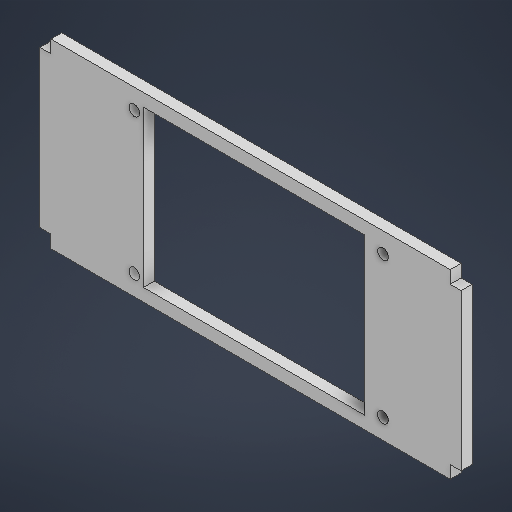
# Autodesk Inventor part: pantallaSoport
Saved by Autodesk Inventor 2026 (Build 300175000, 175)
## iProperties
Created: 2026-04-21
Part Number: pantallaSoport
Material: Generic
Document SubType Name: Modeling
Designer: juana
Density: 1 g/cm^3
Appearance: Default
Author: juana
Autodesk Inventor part; units mm, degrees
ref_plane "YZ Plane" through (0, 0, 0) normal (1, 0, 0) x (0, 1, 0)
ref_plane "XZ Plane" through (0, 0, 0) normal (0, 1, 0) x (-1, 0, 0)
ref_plane "XY Plane" through (0, 0, 0) normal (0, 0, 1) x (1, 0, 0)
sketch "Sketch1" plane through (0, 0, 0) normal (0, 0, 1) x (1, 0, 0)
  line L0 (0, 0) -> (116, 0)
  line L1 (116, 0) -> (116, 50)
  line L2 (116, 50) -> (0, 50)
  line L3 (0, 50) -> (0, 0)
  line L4 (0, 50) -> (3, 50)
  line L5 (3, 50) -> (3, 46.5)
  line L6 (3, 46.5) -> (0, 46.5)
  line L7 (0, 46.5) -> (0, 50)
  line L8 (0, 0) -> (3, 0)
  line L9 (3, 0) -> (3, 3.5)
  line L10 (3, 3.5) -> (0, 3.5)
  line L11 (0, 3.5) -> (0, 0)
  line L12 (58, 0) -> (58, 50) construction
  line L13 (113, 50) -> (113, 46.5)
  line L14 (113, 46.5) -> (116, 46.5)
  line L15 (113, 0) -> (113, 3.5)
  line L16 (113, 3.5) -> (116, 3.5)
  line L17 (19.5, 46.5) -> (96.5, 46.5) construction
  line L18 (96.5, 46.5) -> (96.5, 3.5) construction
  line L19 (96.5, 3.5) -> (19.5, 3.5) construction
  line L20 (19.5, 3.5) -> (19.5, 46.5) construction
  line L21 (28.5, 46.5) -> (89.5, 46.5)
  line L22 (89.5, 46.5) -> (89.5, 3.5)
  line L23 (89.5, 3.5) -> (28.5, 3.5)
  line L24 (28.5, 3.5) -> (28.5, 46.5)
  point P0 (1.5, 25)
  point P1 (0, 25)
  point P2 (1.5, 3.5)
  point P3 (19.5, 25)
  point P4 (58, 46.5)
  point P5 (1.5, 46.5)
  point P6 (94.5, 5.5)
  point P7 (94.5, 44.5)
  point P8 (26, 44.5)
  point P9 (26, 5.5)
  point P10 (0, 46.5)
  point P11 (0, 3.5)
  dimension "d0" = 116
  dimension "d1" = 50
  dimension "d2" = 3
  dimension "d4" = 21.5
  dimension "d5" = 21.5
  dimension "d6" = 77
  dimension "d7" = 61
  dimension "d8" = 9
  dimension "d9" = 2
  dimension "d10" = 2
  dimension "d11" = 2
  dimension "d12" = 6.5
  dimension "d13" = 2
  constraints: 50 end point, 10 parallel, 7 midpoint, 6 horizontal alignment, 6 symmetric about line, 5 horizontal, 5 perpendicular, 5 vertical alignment
  measures "d0" distance of L1.end L2.end
  measures "d1" distance of L0.end L1.end
  measures "d2" distance of L5.end L6.end
  measures "d4" distance from line of L10 point (1.5, 25)
  measures "d5" distance from line of L6 point (1.5, 25)
  measures "d6" distance of L17.start L17.end
  measures "d7" distance of L21.start L21.end
  measures "d8" distance between parallel lines of L20 L24
  measures "d9" distance from line of L19 point (94.5, 5.5)
  measures "d10" distance from line of L17 point (94.5, 44.5)
  measures "d11" distance from line of L18 point (94.5, 44.5)
  measures "d12" distance from line of L20 point (26, 44.5)
  measures "d13" distance from line of L19 point (26, 5.5)
extrude "Extrusion1" add sketch "Sketch1" along normal blind 3 contours L9 L10 L3 L6 L5 L2 L13 L14 L1 L16 L15 L0
sketch "Sketch2" plane through (0, 0, 3) normal (0, 0, 1) x (1, 0, 0)
  line L0 (28.5, 46.5) -> (89.5, 46.5) projected
  line L1 (19.5, 46.5) -> (96.5, 46.5)
  line L2 (96.5, 46.5) -> (96.5, 3.5)
  line L3 (96.5, 3.5) -> (19.5, 3.5)
  line L4 (19.5, 3.5) -> (19.5, 46.5)
  line L5 (113, 50) -> (3, 50) projected
  line L6 (0, 46.5) -> (0, 3.5) projected
  point P0 (0, 0)
  point P1 (25.9672, 44.5)
  point P2 (25.9672, 5.5258)
  point P3 (99.0449, 5.5258)
  point P4 (105.2369, 44.803)
  point P5 (58, 46.5)
  point P6 (58, 50)
  point P7 (19.5, 25)
  point P8 (0, 25)
  point P9 (94.5, 44.5)
  point P10 (94.5, 5.5)
  dimension "d16" = 2
  dimension "d17" = 77
  dimension "d18" = 2
  dimension "d19" = 2
  dimension "d20" = 2
  constraints: 8 end point, 4 midpoint, 3 vertical alignment, 2 parallel, 1 horizontal, 1 horizontal alignment, 1 perpendicular, 1 point on line
  measures "d16" distance from line of L1 point (25.967, 44.5)
  measures "d17" distance between parallel lines of L2 L4
  measures "d18" distance from line of L1 point (94.5, 44.5)
  measures "d19" distance from line of L3 point (94.5, 5.5)
  measures "d20" distance from line of L2 point (94.5, 5.5)
hole "Hole1" at (25.9672, 44.5, 3) at (25.9672, 5.5258, 3) at (94.5, 5.5, 3) at (94.5, 44.5, 3) direction (0, 0, -1) diameter 3 end through all
body "Solid1"
